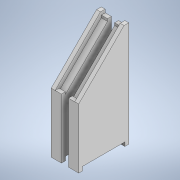
# Autodesk Inventor part: BeamSplitter_Base
Saved by Autodesk Inventor 2022.2 (Build 262287010, 287A)
## iProperties
Created: 2022-03-23
Part Number: BeamSplitter_Base
Material: Genérico
Document SubType Name: Modeling
Designer: mabel
Density: 1 g/cm^3
Appearance: Valor por defecto
Author: mabel
Autodesk Inventor part; units mm, degrees
ref_plane "YZ Plane" through (0, 0, 0) normal (1, 0, 0) x (0, 1, 0)
ref_plane "XZ Plane" through (0, 0, 0) normal (0, 1, 0) x (-1, 0, 0)
sketch "Boceto1" plane through (0, 0, 0) normal (1, 0, 0) x (0, 1, 0)
  line L0 (0, 0) -> (100, 0) construction
  line L1 (0, 0) -> (0, -26.87) construction
  line L2 (0, 0) -> (0, 26.87) construction
  line L3 (100, 0) -> (126.8701, -26.8701) construction
  line L4 (100, 0) -> (138, 0) construction
  line L5 (100, 0) -> (73.1299, 26.8701) construction
  line L6 (100, 0) -> (138, 0) construction
  line L7 (73.1299, 26.8701) -> (126.8701, -26.8701)
  line L8 (0, 26.87) -> (0, -26.87)
  line L9 (73.13, 26.87) -> (76.13, 26.87)
  line L10 (76.13, 26.87) -> (76.13, 31.87)
  line L11 (76.13, 31.87) -> (0, 31.87)
  line L12 (0, 31.87) -> (0, 26.87)
  line L13 (126.87, -26.87) -> (129.87, -26.87)
  line L14 (129.87, -26.87) -> (129.87, -31.87)
  line L15 (129.87, -31.87) -> (0, -31.87)
  line L16 (0, -31.87) -> (0, -26.87)
  constraints: 34 end point, 5 horizontal, 4 parallel, 3 vertical, 2 equal length, 2 perpendicular, 2 point on line
extrude "Extrusión1" add sketch "Boceto1" along normal blind 8
sketch "Boceto2" plane through (8, 0, 0) normal (1, 0, 0) x (0, 0, -1)
  line L0 (-26.87, 76.13) -> (-31.87, 76.13) construction
  line L1 (-31.87, 76.13) -> (-26.87, 76.13)
  line L2 (26.87, 126.87) -> (26.87, 129.87)
  line L3 (31.87, 129.87) -> (26.87, 129.87) projected
  line L4 (26.87, 129.87) -> (31.87, 129.87)
  line L5 (-31.87, 76.13) -> (-26.87, 76.13) construction
  line L6 (25.87, 133.87) -> (31.87, 133.87) construction
  line L7 (31.87, 133.87) -> (31.87, 129.87) construction
  line L8 (-31.87, 76.13) -> (25.87, 133.87)
  line L9 (31.87, 133.87) -> (31.87, 129.87)
  line L10 (25.87, 133.87) -> (31.87, 133.87)
  line L11 (-26.87, 73.13) -> (-26.87, 76.13) projected
  line L12 (-26.87, 76.13) -> (-31.87, 76.13)
  line L13 (-31.87, 76.13) -> (-31.87, 0) projected
  line L14 (-31.87, 76.13) -> (-31.87, 0)
  line L15 (-31.87, 0) -> (31.87, 0) projected
  line L16 (-31.87, 0) -> (31.87, 0)
  line L17 (31.87, 0) -> (31.87, 133.87)
  point P0 (0, 0)
  dimension "d18" = 133.87
  constraints: 26 end point, 3 collinear, 3 horizontal, 2 perpendicular, 2 vertical, 1 point on line
  measures "d18" distance of L15.end L6.end
extrude "Extrusión2" add sketch "Boceto2" along normal blind 5
ref_plane "Plano de trabajo1" through (-4.5, 0, 0) normal (-1, 0, 0) x (0, 0, 1)
mirror "Simetría1" about plane through (-4.5, 0, 0) normal (-1, 0, 0) of "Extrusión1", "Extrusión2"
sketch "Boceto4" plane through (13, 0, 0) normal (1, 0, 0) x (0, 0, -1)
  line L0 (-31.87, 76.13) -> (-31.87, 0) projected
  line L1 (-31.87, 0) -> (-26.87, 0)
  line L2 (-31.87, 0) -> (31.87, 0) projected
  line L3 (-26.87, 0) -> (-26.87, 5)
  line L4 (31.87, 0) -> (26.87, 0)
  line L5 (26.87, 0) -> (26.87, 5)
  line L6 (26.87, 5) -> (-26.87, 5)
  point P0 (0, 0)
  dimension "d23" = 5
  dimension "d24" = 5
  dimension "d25" = 5
  constraints: 10 end point, 2 perpendicular, 2 point on line, 1 vertical
  measures "d23" distance of L0.end L1.end
  measures "d24" distance of L1.end L3.end
  measures "d25" distance of L2.end L4.end
extrude "Extrusión3" cut sketch "Boceto4" against normal through all
